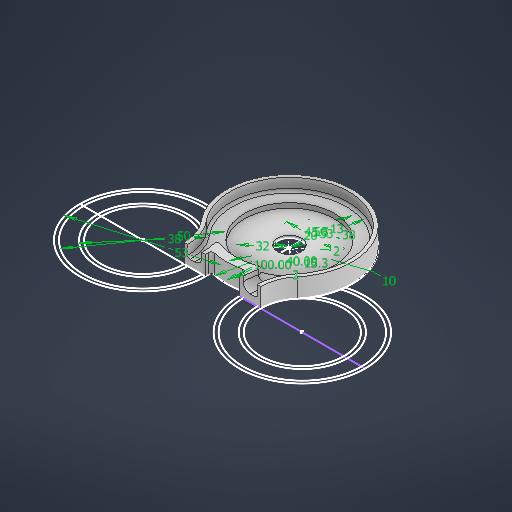
# Autodesk Inventor part: Gehäuse
Saved by Autodesk Inventor 2026.2 (Build 302298000, 298)
## iProperties
Created: 2026-03-18
Part Number: Gehäuse
Material: Generic
Document SubType Name: Modeling
Designer: Cobble
Density: 1 g/cm^3
Appearance: Default
Author: Cobble
Autodesk Inventor part; units mm, degrees
ref_plane "YZ Plane" through (0, 0, 0) normal (1, 0, 0) x (0, 1, 0)
ref_plane "XZ Plane" through (0, 0, 0) normal (0, 1, 0) x (-1, 0, 0)
ref_plane "XY Plane" through (0, 0, 0) normal (0, 0, 1) x (1, 0, 0)
sketch "Sketch1" plane through (0, 0, 0) normal (0, 0, 1) x (1, 0, 0)
  circle A0 centre (0, 0) radius 19
  circle A1 centre (0, 0) radius 16 construction
  circle A2 centre (0, 16) radius 6.5 construction
  circle A3 centre (0, 0) radius 25
  circle A4 centre (0, 0) radius 26.5
  line L0 (0, 0) -> (20.3002, -17.0339)
  line L1 (0, 0) -> (26.5, 0) construction
  line L2 (0, 0) -> (-20.3002, -17.0339)
  line L3 (0, 0) -> (26.5, 0) construction
  circle A5 centre (-33.706, -28.2827) radius 25
  circle A6 centre (-33.706, -28.2827) radius 19
  circle A7 centre (-33.706, -28.2827) radius 17.5
  circle A8 centre (-33.706, -28.2827) radius 26.5
  line L4 (-60.206, -28.2827) -> (-7.206, -28.2827)
  line L5 (0, -16) -> (0, 16)
  circle A9 centre (33.706, -28.2827) radius 25
  circle A10 centre (33.706, -28.2827) radius 19
  circle A11 centre (33.706, -28.2827) radius 17.5
  circle A12 centre (33.706, -28.2827) radius 26.5
  circle A13 centre (0, 0) radius 5
  line L6 (60.206, -28.2827) -> (7.206, -28.2827)
  circle A14 centre (0, 0) radius 22.75
  line L7 (-10, -7.65) -> (10, -7.65)
  line L8 (10, -7.65) -> (10, 7.65)
  line L9 (10, 7.65) -> (-10, 7.65)
  line L10 (-10, 7.65) -> (-10, -7.65)
  line L11 (-10, -7.65) -> (10, 7.65) construction
  line L12 (10, -7.65) -> (-10, 7.65) construction
  line L13 (-10, -7.65) -> (10, -7.65)
  line L14 (10, -7.65) -> (10, -9.65)
  line L15 (10, -9.65) -> (-10, -9.65)
  line L16 (-10, -9.65) -> (-10, -7.65)
  line L17 (-10, 7.65) -> (10, 7.65)
  line L18 (10, 7.65) -> (10, 9.65)
  line L19 (10, 9.65) -> (-10, 9.65)
  line L20 (-10, 9.65) -> (-10, 7.65)
  point P0 (-14.5548, -12.213)
  point P1 (-8.706, -28.2827)
  point P2 (-7.3569, -25.4583)
  point P3 (7.3569, -25.4583)
  point P4 (8.706, -28.2827)
  point P5 (14.5548, -12.213)
  point P6 (-16.206, -28.2827)
  point P7 (-14.706, -28.2827)
  point P8 (-19.1511, -16.0697)
  point P9 (19.1511, -16.0697)
  point P10 (14.706, -28.2827)
  point P11 (16.206, -28.2827)
  point P12 (-9.2203, -23.2376)
  point P13 (9.2203, -23.2376)
  point P14 (9.964, -20.4519)
  point P15 (-9.964, -20.4519)
  dimension "d10" = 53
  dimension "d1" = 32
  dimension "d2" = 13
  dimension "d3" = 50
  dimension "d4" = 53
  dimension "d5" = 38
  dimension "d6" = 40
  dimension "d8" = 50
  dimension "d9" = 38
  dimension "d11" = 100
  dimension "d12" = 10
  dimension "d20" = 45.5
  dimension "d23" = 20
  dimension "d24" = 15.3
  dimension "d25" = 2
  dimension "d26" = 2
  constraints: 42 end point, 12 centre point, 12 coincident, 6 horizontal, 6 parallel, 5 midpoint, 4 perpendicular, 4 point on circle, 4 symmetric about line, 2 equal length, 1 line through centre, 1 point on line, 1 tangent, 1 vertical, 12 other
  measures "d1" diameter of A1
  measures "d2" diameter of A2
  measures "d3" diameter of A3
  measures "d4" diameter of A4
  measures "d5" diameter of A0
  measures "d6" angle of L0 L1
  measures "d8" diameter of A5
  measures "d9" diameter of A6
  measures "d11" angle of L0 L2
  measures "d12" diameter of A13
  measures "d20" diameter of A14
  measures "d23" distance of L9.end L8.end
  measures "d24" distance of L8.end L7.end
  measures "d25" distance of L13.end L14.end
  measures "d26" distance of L18.end L17.end
extrude "Extrusion1" add sketch "Sketch1" along normal blind 8 contours A14 A8 A3 A5 | A8 A4 A12 A3 | A3 A5 A4 A8 | A9 A3 A12 A14 | A12 A4 A9 A3 | A14 A12 A3 A8 | A6 A4 A5 A3 | A6 A4 L2 | L2 A4 A6 | A3 A8 A4 A5 | A10 A4 L0 | A3 A9 A4 A10 | L0 A4 A10 | A9 A4 A12 A3 | A3 A12 A4 A8 | A4 A6 L4 A7 | A4 A8 L4 A5 | A11 L6 A10 A4 | A9 L6 A12 A4 picked at (-8.6838, -22.6121) picked at (8.6838, -22.6121) picked at (0.8547, -23.3428) picked at (-24.4427, -7.0635) picked at (24.4427, -7.0635) picked at (-15.9175, -26.1102) picked at (-8.2697, -26.5414) picked at (15.9175, -26.1102) picked at (8.2697, -26.5414)
extrude "Extrusion2" add sketch "Sketch1" along normal blind 3 contours A0 A8 A14 A12 | A0 A5 A14 A8 | A12 A14 A9 A0 | A5 A14 L2 | A0 A8 A14 A5 | L2 A14 A5 | A14 A5 A3 A8 | A8 A3 A12 A14 | A9 A14 A12 A0 | A9 A14 L0 | L0 A14 A9 | A12 A3 A9 A14 | A0 A12 A14 A8 | A14 A5 A3 L2 | L2 A3 A5 A14 | A14 A9 A3 L0 | L0 A3 A9 A14 | A3 A5 A4 A6 | A10 A4 A9 A3 | A4 A5 L4 A6 | A10 L6 A9 A4 picked at (-23.7765, -4.6253) picked at (24.023, 1.9318) picked at (23.7765, -4.6253) picked at (-11.2006, -22.8448) picked at (11.2006, -22.8448) picked at (-11.6356, -26.4469) picked at (11.6356, -26.4469)
extrude "Extrusion3" add sketch "Sketch1" along normal blind 1 contours A0 A12 L0 L14 L8 L18 L19 L20 L10 L16 L2 A8 | A8 L2 A0 | A0 L0 A12 | L2 A8 A0 | L2 L16 L15 L14 L0 A12 A0 A8 | A0 A12 L0 | L16 L7 L2 | L2 L7 L5 L15 L16 | L14 L15 L5 L7 L0 | L0 L7 L14 | L7 L10 L9 L5 A13 L2 | L2 A13 L5 L7 | L7 L5 A13 L0 | L0 A13 L5 L9 L8 L7 | L20 L19 L5 L9 | L9 L5 L19 L18
fillet "Fillet1" radius 1 3 edges at (15.8518, -21.7843, 3) (-15.8518, -21.7843, 3) (0, 25, 3)
fillet "Fillet2" radius 3 2 edges at (-9.0225, -24.3171, 3) (9.0225, -24.3171, 3)
fillet "Fillet3" radius 1 6 edges at (-11.4563, -19.6549, 3.6493) (-9.964, -20.4519, 7) (11.4563, -19.6549, 3.6493) (9.964, -20.4519, 7) (-7.3569, -25.4583, 4) (7.3569, -25.4583, 4)
body "Solid1"
